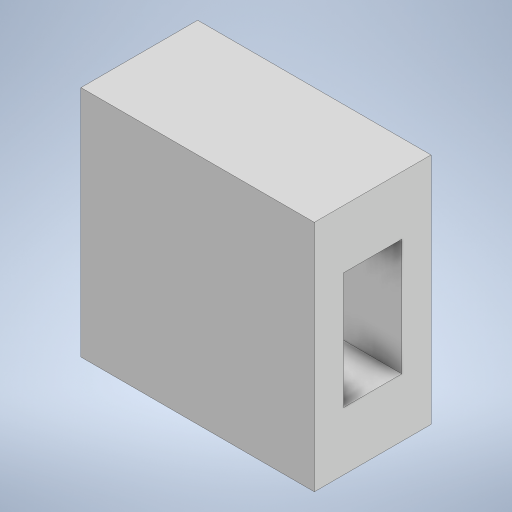
# Autodesk Inventor part: goi truot
Saved by Autodesk Inventor 2024 (Build 280153000, 153)
## iProperties
Created: 2025-09-18
Part Number: goi truot
Material: Generic
Document SubType Name: Modeling
Designer: Hello
Density: 1 g/cm^3
Appearance: Default
Author: Hello
Autodesk Inventor part; units mm, degrees
ref_plane "YZ Plane" through (0, 0, 0) normal (1, 0, 0) x (0, 1, 0)
ref_plane "XZ Plane" through (0, 0, 0) normal (0, 1, 0) x (-1, 0, 0)
ref_plane "XY Plane" through (0, 0, 0) normal (0, 0, 1) x (1, 0, 0)
sketch "Sketch1" plane through (0, 0, 0) normal (0, 0, 1) x (1, 0, 0)
  line L0 (0, 0) -> (40, 0)
  line L1 (40, 0) -> (40, 40)
  line L2 (0, 40) -> (0, 0)
  line L3 (0, 40) -> (40, 40)
  dimension "d0" = 40
  dimension "d1" = 40
  constraints: 8 end point, 2 horizontal, 1 parallel, 1 perpendicular
  measures "d0" distance of L2.start L0.start
  measures "d1" distance of L0.start L0.end
extrude "Extrusion1" add sketch "Sketch1" along normal blind 20
sketch "Sketch2" plane through (40, 0, 0) normal (1, 0, 0) x (0, 0, -1)
  line L0 (-15, 30) -> (-5, 30)
  line L1 (-5, 30) -> (-5, 10)
  line L2 (-5, 10) -> (-15, 10)
  line L3 (-15, 10) -> (-15, 30)
  line L4 (-20, 0) -> (-20, 40) projected
  line L5 (0, 0) -> (-20, 0) projected
  dimension "d7" = 20
  dimension "d8" = 10
  dimension "d9" = 5
  dimension "d10" = 10
  constraints: 8 end point, 2 parallel, 1 horizontal, 1 perpendicular
  measures "d7" distance of L2.end L0.start
  measures "d8" distance of L1.end L2.end
  measures "d9" distance between parallel lines of L4 L3
  measures "d10" distance between parallel lines of L2 L5
extrude "Extrusion2" cut sketch "Sketch2" against normal through all
body "Solid1"
